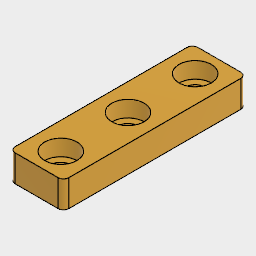
Belt_Clamp_F01 (Autodesk Fusion 360 design; units mm, degrees)
Autodesk Fusion 360 part; units mm, degrees
sketch "スケッチ1" plane through (0, 0, 0) normal (0, 0, 1) x (1, 0, 0)
  line L0 (0, 0) -> (10, 0)
  line L1 (10, 0) -> (10, 34)
  line L2 (10, 34) -> (0, 34)
  line L3 (0, 34) -> (0, 0)
  line L4 (5, 34) -> (5, 0) construction
  line L5 (0, 17) -> (10, 17) construction
  circle A0 centre (5, 17) radius 1.75
  circle A1 centre (5, 29.5) radius 1.75
  circle A2 centre (5, 4.5) radius 1.75
  dimension "d1" = 34
  dimension "d2" = 10
  dimension "d3" = 3.5
  dimension "d4" = 3.5
  dimension "d5" = 3.5
  dimension "d6" = 12.5
  dimension "d7" = 12.5
  measures "d1" distance of L0.start L2.end
  measures "d2" distance of L0.start L0.end
  measures "d3" diameter of A1
  measures "d4" diameter of A0
  measures "d5" diameter of A2
  measures "d6" distance of A0.centre A1.centre
  measures "d7" distance of A0.centre A2.centre
extrude "押し出し1" add sketch "スケッチ1" along normal blind 5
sketch "スケッチ2" plane through (0, 0, 5) normal (0, 0, 1) x (-1, 0, 0)
  circle A0 centre (-5, -4.5) radius 1.75
  circle A1 centre (-5, -29.5) radius 1.75
  circle A2 centre (-5, -17) radius 1.75
  line L0 (0, -34) -> (0, 0)
  line L1 (0, 0) -> (-10, 0)
  line L2 (-10, 0) -> (-10, -34)
  line L3 (-10, -34) -> (0, -34)
  circle A3 centre (-5, -29.5) radius 3
  circle A4 centre (-5, -17) radius 3
  circle A5 centre (-5, -4.5) radius 3
  dimension "d10" = 6
  dimension "d11" = 6
  dimension "d12" = 6
  measures "d10" diameter of A3
  measures "d11" diameter of A4
  measures "d12" diameter of A5
extrude "押し出し2" cut sketch "スケッチ2" against normal blind 3 contours A3 | A4 | A5
fillet "フィレット1" radius 1 4 edges at (0, 0, 2.5) (10, 0, 2.5) (10, 34, 2.5) (0, 34, 2.5)
